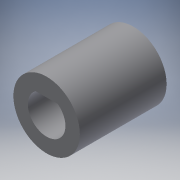
# Autodesk Inventor part: NewDriveWheel2
Saved by Autodesk Inventor 2019 (Build 230136000, 136)
## iProperties
Created: 2021-11-20
Part Number: NewDriveWheel2
Material: Generic
Document SubType Name: Modeling
Designer: Ian
Density: 1 g/cm^3
Appearance: Default
Author: Ian
Autodesk Inventor part; units mm, degrees
ref_plane "YZ Plane" through (0, 0, 0) normal (1, 0, 0) x (0, 1, 0)
ref_plane "XZ Plane" through (0, 0, 0) normal (0, 1, 0) x (-1, 0, 0)
ref_plane "XY Plane" through (0, 0, 0) normal (0, 0, 1) x (1, 0, 0)
sketch "Sketch1" plane through (0, 0, 0) normal (0, 0, 1) x (1, 0, 0)
  line L0 (1.5, 2) -> (-1.5, 2) construction
  arc A0 (-1.5, 2) -> (1.5, 2) centre (0, 0) ccw construction
  circle A1 centre (0, 0) radius 11 construction
  arc A2 (-1.5, 2) -> (1.5, 2) centre (0, 0) ccw construction
  line L1 (1.5, 2) -> (-1.5, 2) construction
  circle A3 centre (0, 0) radius 4.6
  arc A4 (-1.533, 2.1) -> (1.533, 2.1) centre (0, 0) ccw
  line L2 (-1.533, 2.1) -> (1.533, 2.1)
  dimension "d0" = 9.2
  dimension "d1" = 5.2
  dimension "d2" = 0.1
  constraints: 2 centre point, 2 coincident, 2 end point, 2 point on circle, 1 horizontal
  measures "d0" diameter of A3
  measures "d1" diameter of A4
  measures "d2" distance between parallel lines of L0 L2
extrude "Extrusion1" add sketch "Sketch1" along normal blind 12
sketch "Sketch2" plane through (0, 0, 0) normal (1, 0, 0) x (0, 1, 0)
  line L0 (0, 12.2) -> (21, 12.2) construction
  line L1 (8.4705, 1) -> (21, 1) construction
  line L2 (0, -2.44) -> (0, 14.64) projected
  line L3 (4.6, 0) -> (4.6, 12) construction
  line L4 (4.6, 10.36) -> (3.8845, 10.36) construction
  line L5 (4.6, 0) -> (4.6, 12) construction
  line L6 (4.6, 9.56) -> (3.8621, 9.56) construction
  line L7 (4.6, 10.36) -> (4, 10.04)
  line L8 (4, 10.04) -> (4, 9.88)
  line L9 (4.6, 0) -> (4.6, 12) construction
  line L10 (4, 9.88) -> (4.6, 9.56)
  line L11 (4.6, 9.56) -> (4.6, 9.4)
  line L12 (4.6, 0) -> (4.6, 12) construction
  line L13 (4.6, 9.4) -> (4, 9.08)
  line L14 (4, 9.08) -> (4, 8.92)
  line L15 (4, 8.92) -> (4.6, 8.6)
  line L16 (4.6, 8.6) -> (4.6, 8.44)
  line L17 (4.6, 8.44) -> (4, 8.12)
  line L18 (4, 8.12) -> (4, 7.96)
  line L19 (4, 7.96) -> (4.6, 7.64)
  line L20 (4.6, 7.64) -> (4.6, 7.48)
  line L21 (4.6, 7.48) -> (4, 7.16)
  line L22 (4, 7.16) -> (4, 7)
  line L23 (4, 7) -> (4.6, 6.68)
  line L24 (4.6, 6.68) -> (4.6, 6.52)
  line L25 (4.6, 6.52) -> (4, 6.2)
  line L26 (4, 6.2) -> (4, 6.04)
  line L27 (4, 6.04) -> (4.6, 5.72)
  line L28 (4.6, 5.72) -> (4.6, 5.56)
  line L29 (4.6, 5.56) -> (4, 5.24)
  line L30 (4, 5.24) -> (4, 5.08)
  line L31 (4, 5.08) -> (4.6, 4.76)
  line L32 (4.6, 4.76) -> (4.6, 4.6)
  line L33 (4.6, 4.6) -> (4, 4.28)
  line L34 (4, 4.28) -> (4, 4.12)
  line L35 (4, 4.12) -> (4.6, 3.8)
  line L36 (4.6, 3.8) -> (4.6, 3.64)
  line L37 (4.6, 3.64) -> (4, 3.32)
  line L38 (4, 3.32) -> (4, 3.16)
  line L39 (4, 3.16) -> (4.6, 2.84)
  line L40 (4.6, 2.84) -> (4.6, 2.68)
  line L41 (4.6, 10.36) -> (4.6, 12.2) construction
  line L42 (4.6, 10.36) -> (6.2592, 10.36) construction
  line L43 (6.2592, 10.36) -> (6.2592, 12.2) construction
  line L44 (4.6, 2.84) -> (5.8943, 2.84) construction
  line L45 (5.8943, 2.84) -> (5.8943, 1) construction
  line L46 (4.6, 10.36) -> (4.6, 9.56)
  line L47 (4.6, 9.4) -> (4.6, 8.6)
  line L48 (4.6, 8.44) -> (4.6, 7.64)
  line L49 (4.6, 7.48) -> (4.6, 6.68)
  line L50 (4.6, 0) -> (4.6, 12) projected
  line L51 (4.6, 6.52) -> (4.6, 5.72)
  line L52 (4.6, 0) -> (4.6, 12) projected
  line L53 (4.6, 5.56) -> (4.6, 4.76)
  line L54 (4.6, 4.6) -> (4.6, 3.8)
  line L55 (4.6, 0) -> (4.6, 12) projected
  line L56 (4.6, 3.64) -> (4.6, 2.84)
  line L57 (4.6, 0) -> (4.6, 12) projected
  point P0 (0, 0)
  dimension "d6" = 0.8
  dimension "d7" = 0.16
  dimension "d8" = 0.6
  dimension "d9" = 0.16
  dimension "d12" = 0.96
  constraints: 94 end point, 35 vertical alignment, 16 collinear, 15 parallel, 5 vertical, 4 point on line, 3 horizontal, 3 perpendicular, 2 equal length, 10 other
  measures "d6" distance between parallel lines of L4 L6
  measures "d7" distance of L7.end L8.end
  measures "d9" distance of L6.start L11.end
  measures "d12" distance of L4.start L13.start
revolve "Revolution1" cut sketch "Sketch2" angle 360 about axis through (0, 0, -10) along (0, 0, 1)
sketch "Sketch3" plane through (0, 0, 0) normal (0, 0, -1) x (-1, 0, 0)
  circle A0 centre (0, 0) radius 4.6 projected
  circle A1 centre (0, 0) radius 6.6
  dimension "d17" = 2
  constraints: 1 centre point
  measures "d17" radial gap between concentric circles of A0 A1
extrude "Extrusion2" add sketch "Sketch3" against normal blind 1
body "Solid1"
